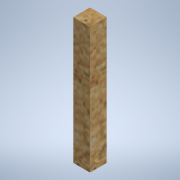
# Autodesk Inventor part: Adrian_Cameraarmseiten
Saved by Autodesk Inventor 2021 (Build 250183000, 183)
## iProperties
Created: 2022-07-12
Part Number: Adrian_Cameraarmseiten
Material: Generisch
Document SubType Name: Modeling
Designer: adria
Mass: 475.947 g
Surface Area: 524.189 cm^2
Volume: 475.947 cm^3
Density: 1 g/cm^3
Appearance: Vorgabe
Author: adria
Autodesk Inventor part; units mm, degrees
ref_plane "YZ Plane" through (0, 0, 0) normal (1, 0, 0) x (0, 1, 0)
ref_plane "XZ Plane" through (0, 0, 0) normal (0, 1, 0) x (-1, 0, 0)
ref_plane "XY Plane" through (0, 0, 0) normal (0, 0, 1) x (1, 0, 0)
sketch "Skizze1" plane through (0, 0, 0) normal (0, 1, 0) x (-1, 0, 0)
  line L0 (-20, 20) -> (20, 20)
  line L1 (20, 20) -> (20, -20)
  line L2 (20, -20) -> (-20, -20)
  line L3 (-20, -20) -> (-20, 20)
  line L4 (-20, 20) -> (20, -20) construction
  line L5 (20, 20) -> (-20, -20) construction
  point P0 (0, 0)
  dimension "d2" = 40
  dimension "d3" = 40
  constraints: 12 end point, 2 midpoint, 2 parallel, 1 horizontal, 1 perpendicular
  measures "d2" distance of L1.end L2.end
  measures "d3" distance of L0.end L1.end
extrude "Extrusion1" add sketch "Skizze1" along normal blind 300
sketch "Skizze2" plane through (20, 0, 20) normal (1, 0, 0) x (0, 0, -1)
  line L0 (0, 0) -> (40, 0) projected
  point P0 (20, 0)
  point P1 (20, 20)
  point P2 (20, 0)
  dimension "d4" = 20
  constraints: 1 midpoint, 1 vertical alignment
  measures "d4" distance from line of point (20, 20) L0
hole "Bohrung1" at (20, 20, 0) direction (-1, 0, 0) diameter 8 end through all counterbore diameter 18 counterbore depth 10
equation "\"d3\" = d2"
